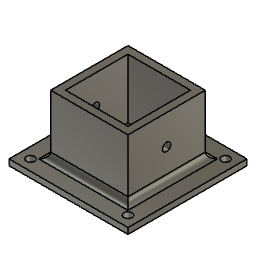
Flange v3 v5 (Autodesk Fusion 360 design; units mm, degrees)
Autodesk Fusion 360 part; units mm, degrees
sketch "Sketch1" plane through (0, 0, 0) normal (0, 0, 1) x (1, 0, 0)
  line L0 (13.335, 13.335) -> (-13.335, 13.335)
  line L1 (-13.335, 13.335) -> (-13.335, -13.335)
  line L2 (-13.335, -13.335) -> (13.335, -13.335)
  line L3 (13.335, -13.335) -> (13.335, 13.335)
  line L4 (13.335, 13.335) -> (-13.335, -13.335) construction
  line L5 (-13.335, 13.335) -> (13.335, -13.335) construction
  line L6 (16.51, 16.51) -> (-16.51, 16.51)
  line L7 (-16.51, 16.51) -> (-16.51, -16.51)
  line L8 (-16.51, -16.51) -> (16.51, -16.51)
  line L9 (16.51, -16.51) -> (16.51, 16.51)
  line L10 (16.51, 16.51) -> (-16.51, -16.51) construction
  line L11 (-16.51, 16.51) -> (16.51, -16.51) construction
  dimension "d1" = 26.67
  dimension "d2" = 26.67
  dimension "d3" = 33.02
  dimension "d4" = 33.02
  constraint horizontal L0
  constraint perpendicular L0 L1
  constraint parallel L0 L2
  constraint parallel L1 L3
  constraint coincident L4 origin
  constraint coincident L5 origin
  constraint horizontal L6
  constraint perpendicular L6 L7
  constraint parallel L6 L8
  constraint parallel L7 L9
  constraint coincident L10 origin
  constraint coincident L11 origin
  measures "d1" distance of L0.start L0.end
  measures "d2" distance of L2.end L0
  measures "d3" distance of L7.end L8.end
  measures "d4" distance of L6.start L8.end
extrude "Extrude1" add sketch "Sketch1" along normal blind 25.4
sketch "Sketch2" plane through (0, 0, 0) normal (0, 0, 1) x (1, 0, 0)
  line L0 (25.4, 25.4) -> (-25.4, 25.4)
  line L1 (-25.4, 25.4) -> (-25.4, -25.4)
  line L2 (-25.4, -25.4) -> (25.4, -25.4)
  line L3 (25.4, -25.4) -> (25.4, 25.4)
  line L4 (25.4, 25.4) -> (-25.4, -25.4) construction
  line L5 (-25.4, 25.4) -> (25.4, -25.4) construction
  dimension "d7" = 50.8
  dimension "d8" = 50.8
  constraint horizontal L0
  constraint perpendicular L0 L1
  constraint parallel L0 L2
  constraint parallel L1 L3
  constraint coincident L4 origin
  constraint coincident L5 origin
  measures "d7" distance of L1.end L2.end
  measures "d8" distance of L0.end L1.end
extrude "Extrude2" add sketch "Sketch2" against normal blind 2.54
fillet "Fillet1" radius 2.54 4 edges at (16.51, 0, 0) (0, -16.51, 0) (-16.51, 0, 0) (0, 16.51, 0)
sketch "Sketch4" plane through (0, 0, 0) normal (0, 0, 1) x (-1, 0, 0)
  line L0 (-25.4, 25.4) -> (-25.4, -25.4)
  line L1 (-25.4, -25.4) -> (25.4, -25.4)
  line L2 (25.4, -25.4) -> (25.4, 25.4)
  line L3 (25.4, 25.4) -> (-25.4, 25.4)
  line L4 (-19.05, -19.05) -> (-19.05, 19.05)
  line L5 (-19.05, 19.05) -> (19.05, 19.05)
  line L6 (19.05, 19.05) -> (19.05, -19.05)
  line L7 (19.05, -19.05) -> (-19.05, -19.05)
  circle A0 centre (20.828, -20.828) radius 1.778
  circle A1 centre (-20.828, -20.828) radius 1.778
  circle A2 centre (20.828, 20.828) radius 1.778
  circle A3 centre (-20.828, 20.828) radius 1.778
  dimension "d14" = 3.556
  dimension "d15" = 3.556
  dimension "d16" = 3.556
  dimension "d17" = 3.556
  dimension "d18" = 4.572
  dimension "d19" = 4.572
  dimension "d20" = 4.572
  dimension "d21" = 4.572
  dimension "d22" = 4.572
  dimension "d23" = 4.572
  dimension "d25" = 4.572
  dimension "d41" = 4.572
  measures "d14" diameter of A0
  measures "d15" diameter of A1
  measures "d16" diameter of A2
  measures "d17" diameter of A3
  measures "d18" distance of L2 A0.centre
  measures "d19" distance of L1 A0.centre
  measures "d20" distance of L1 A1.centre
  measures "d21" distance of L0 A1.centre
  measures "d22" distance of L2 A2.centre
  measures "d23" distance of L3 A2.centre
  measures "d25" distance of L3 A3.centre
  measures "d41" distance of L0 A3.centre
extrude "Extrude3" cut sketch "Sketch4" against normal blind 2.54 contours A0 | A1 | A2 | A3
sketch "Sketch5" plane through (-16.51, 0, 0) normal (-1, 0, 0) x (0, -1, 0)
  line L0 (-16.51, 2.54) -> (16.51, 2.54)
  line L1 (16.51, 2.54) -> (16.51, 25.4)
  line L2 (16.51, 25.4) -> (-16.51, 25.4)
  line L3 (-16.51, 25.4) -> (-16.51, 2.54)
  circle A0 centre (0.6022, 12.7) radius 1.778
  dimension "d28" = 3.556
  dimension "d29" = 12.7
  dimension "d30" = 15.9078
  measures "d28" diameter of A0
  measures "d29" distance of L2 A0.centre
  measures "d30" distance of L1 A0.centre
extrude "Extrude4" cut sketch "Sketch5" against normal blind 5.08 contours A0
sketch "Sketch7" plane through (16.51, 0, 0) normal (1, 0, 0) x (0, 1, 0)
  line L0 (-16.51, 2.54) -> (16.51, 2.54)
  line L1 (16.51, 2.54) -> (16.51, 25.4)
  line L2 (16.51, 25.4) -> (-16.51, 25.4)
  line L3 (-16.51, 25.4) -> (-16.51, 2.54)
  circle A0 centre (-0.0337, 12.7) radius 1.778
  dimension "d37" = 3.556
  dimension "d38" = 12.7
  measures "d37" diameter of A0
  measures "d38" distance of L2 A0.centre
extrude "Extrude6" cut sketch "Sketch7" against normal blind 5.08 contours A0
